Test+Gear (Autodesk Fusion 360 design; units mm, degrees)
Autodesk Fusion 360 part; units mm, degrees
sketch "Sketch1" plane through (0, 0, 0) normal (0, 0, 1) x (1, 0, 0) in component "Component"
  line L0 (0, 0) -> (2.9094, 11.25)
  line L1 (8.1773, 11.25) -> (11.0867, 0)
  line L2 (2.9094, 11.25) -> (8.1773, 11.25)
  line L3 (0, 0) -> (0, -10)
  line L4 (0, -10) -> (11.0867, -10)
  line L5 (11.0867, -10) -> (11.0867, 0)
  line L6 (6.3765, 0) -> (100, 0)
  line L7 (0, 0, 0) -> (0, 0, 10)
sketch "Sketch2" plane through (0, 0, 0) normal (0, 0, 1) x (1, 0, 0) in component "Component"
  line L0 (0, 0) -> (780.7769, 0)
  line L1 (0, 0) -> (0, -10)
  line L2 (0, -10) -> (780.7769, -10)
  line L3 (780.7769, -10) -> (780.7769, 0)
sweep "Sweep1" add kept parallel profiles "Sketch1" path "Sketch1" along L7 section 1 makes body 1 in component "Component"
pattern_path "PathPattern1" count 50 spacing 15.708 from (6.3765, 0, 0) path "Sketch1" along L6 of "Sweep1" makes body 2 makes body 3 makes body 4 makes body 5 makes body 6 makes body 7 makes body 8 makes body 9 makes body 10 makes body 11 makes body 12 makes body 13 makes body 14 makes body 15 makes body 16 makes body 17 makes body 18 makes body 19 makes body 20 makes body 21 makes body 22 makes body 23 makes body 24 makes body 25 makes body 26 makes body 27 makes body 28 makes body 29 makes body 30 makes body 31 makes body 32 makes body 33 makes body 34 makes body 35 makes body 36 makes body 37 makes body 38 makes body 39 makes body 40 makes body 41 makes body 42 makes body 43 makes body 44 makes body 45 makes body 46 makes body 47 makes body 48 makes body 49 makes body 50 in component "Component"
extrude "Extrude1" add sketch "Sketch2" along normal blind 10 bodies 1 2 3 4 5 6 7 8 9 10 11 12 13 14 15 16 17 18 19 20 21 22 23 24 25 26 27 28 29 30 31 32 33 34 35 36 37 38 39 40 41 42 43 44 45 46 47 48 49 50 in component "Component"
move_body "Move1" bodies 1 to x (1, 0, 0) y (0, 0, 1) z (0, -1, 0) at (0, -10, 10) in component "Component"
sketch "Sketch3" plane through (0, 0, 0) normal (0, 0, 1) x (1, 0, 0) in component "Component"
  line L0 (0, 0) -> (46.6318, 0) construction
  line L1 (46.6318, 0) -> (46.6318, 3) construction
  line L2 (46.6318, 3) -> (0, 3) construction
  line L3 (0, 3) -> (0, 0) construction
  constraint perpendicular L0 L1
  constraint parallel L0 L2
  constraint parallel L1 L3
sketch "Sketch1 (2)" plane through (0, 0, 0) normal (0, 0, 1) x (1, 0, 0) in component "Component'"
  spline S0 degree 5 poles (40.9519, -4.0239) (40.9523, -4.0239) (40.9533, -4.024) (40.9549, -4.0241) (40.9574, -4.0243) (40.9613, -4.0246) (40.9658, -4.0249) (40.9709, -4.0253) (40.9766, -4.0256) (40.9828, -4.026) (40.9896, -4.0264) (40.9968, -4.0268) (41.0046, -4.0271) (41.0128, -4.0275) (41.0215, -4.0279) (41.0307, -4.0282) (41.0402, -4.0285) (41.0502, -4.0288) (41.0606, -4.0291) (41.0714, -4.0293) (41.0825, -4.0295) (41.0941, -4.0297) (41.106, -4.0299) (41.1182, -4.03) (41.1308, -4.03) (41.1437, -4.0301) (41.157, -4.0301) (41.1705, -4.03) (41.1844, -4.0299) (41.1986, -4.0297) (41.2131, -4.0295) (41.2279, -4.0293) (41.243, -4.029) (41.2583, -4.0286) (41.274, -4.0282) (41.2899, -4.0278) (41.306, -4.0272) (41.3225, -4.0267) (41.3392, -4.026) (41.3561, -4.0253) (41.3733, -4.0246) (41.3908, -4.0237) (41.4084, -4.0228) (41.4264, -4.0219) (41.4445, -4.0209) (41.4629, -4.0198) (41.4815, -4.0187) (41.5003, -4.0174) (41.5194, -4.0162) (41.5386, -4.0148) (41.5581, -4.0134) (41.5778, -4.0119) (41.5977, -4.0103) (41.6178, -4.0087) (41.6381, -4.007) (41.6586, -4.0052) (41.6793, -4.0034) (41.7002, -4.0014) (41.7212, -3.9994) (41.7425, -3.9974) (41.764, -3.9952) (41.7856, -3.993) (41.8074, -3.9907) (41.8294, -3.9883) (41.8516, -3.9858) (41.8739, -3.9833) (41.8964, -3.9807) (41.9191, -3.978) (41.9419, -3.9752) (41.965, -3.9724) (41.9881, -3.9694) (42.0115, -3.9664) (42.035, -3.9633) (42.0586, -3.9602) (42.0825, -3.9569) (42.1064, -3.9536) (42.1305, -3.9501) (42.1548, -3.9466) (42.1792, -3.9431) (42.2038, -3.9394) (42.2285, -3.9356) (42.2534, -3.9318) (42.2784, -3.9279) (42.3036, -3.9239) (42.3289, -3.9198) (42.3543, -3.9156) (42.3799, -3.9113) (42.4056, -3.907) (42.4314, -3.9025) (42.4574, -3.898) (42.4835, -3.8934) (42.5097, -3.8887) (42.5361, -3.8839) (42.5626, -3.8791) (42.5892, -3.8741) (42.6159, -3.8691) (42.6428, -3.8639) (42.6698, -3.8587) (42.6969, -3.8534) (42.7241, -3.848) (42.7515, -3.8425) (42.779, -3.8369) (42.8066, -3.8313) (42.8343, -3.8255) (42.8621, -3.8197) (42.89, -3.8137) (42.9181, -3.8077) (42.9462, -3.8016) (42.9745, -3.7954) (43.0029, -3.7891) (43.0314, -3.7827) (43.06, -3.7762) (43.0887, -3.7696) (43.1175, -3.763) (43.1464, -3.7562) (43.1754, -3.7494) (43.2045, -3.7424) (43.2337, -3.7354) (43.2631, -3.7283) (43.2925, -3.7211) (43.322, -3.7138) (43.3516, -3.7064) (43.3814, -3.6989) (43.4112, -3.6913) (43.4411, -3.6836) (43.4711, -3.6759) (43.5012, -3.668) (43.5314, -3.66) (43.5617, -3.652) (43.592, -3.6438) (43.6225, -3.6356) (43.653, -3.6273) (43.6837, -3.6189) (43.7144, -3.6103) (43.7452, -3.6017) (43.7762, -3.593) (43.8071, -3.5842) (43.8382, -3.5753) (43.8694, -3.5663) (43.9006, -3.5573) (43.932, -3.5481) (43.9634, -3.5388) (43.9949, -3.5294) (44.0264, -3.52) (44.0581, -3.5104) (44.0898, -3.5008) (44.1216, -3.491) (44.1535, -3.4812) (44.1855, -3.4712) (44.2175, -3.4612) (44.2496, -3.4511) (44.2818, -3.4409) (44.3141, -3.4305) (44.3465, -3.4201) (44.3789, -3.4096) (44.4114, -3.399) (44.4439, -3.3883) (44.4765, -3.3775) (44.5093, -3.3666) (44.542, -3.3556) (44.5749, -3.3445) (44.6078, -3.3333) (44.6408, -3.3221) (44.6738, -3.3107) (44.7069, -3.2992) (44.7401, -3.2877) (44.7733, -3.276) (44.8067, -3.2642) (44.84, -3.2524) (44.8735, -3.2404) (44.907, -3.2284) (44.9405, -3.2162) (44.9742, -3.204) (45.0079, -3.1916) (45.0416, -3.1792) (45.0754, -3.1667) (45.1093, -3.154) (45.1432, -3.1413) (45.1772, -3.1285) (45.2113, -3.1156) (45.2454, -3.1025) (45.2795, -3.0894) (45.3138, -3.0762) (45.348, -3.0629) (45.3824, -3.0495) (45.4168, -3.036) (45.4512, -3.0224) (45.4857, -3.0087) (45.5203, -2.9949) (45.5549, -2.981) (45.5895, -2.967) (45.6242, -2.9529) (45.659, -2.9387) (45.6938, -2.9245) (45.7287, -2.9101) (45.7636, -2.8956) (45.7986, -2.881) (45.8336, -2.8664) (45.8687, -2.8516) (45.9038, -2.8367) (45.9389, -2.8218) (45.9741, -2.8067) (46.0094, -2.7915) (46.0447, -2.7763) (46.0801, -2.7609) (46.1154, -2.7455) (46.1509, -2.7299) (46.1864, -2.7143) (46.2219, -2.6985) (46.2575, -2.6827) (46.2931, -2.6668) (46.3288, -2.6507) (46.3645, -2.6346) (46.4002, -2.6184) (46.436, -2.602) (46.4718, -2.5856) (46.5077, -2.5691) (46.5436, -2.5525) (46.5796, -2.5357) (46.6155, -2.5189) (46.6516, -2.502) (46.6876, -2.485) (46.7237, -2.4679) (46.7599, -2.4507) (46.7961, -2.4334) (46.8323, -2.416) (46.8685, -2.3985) (46.9048, -2.3809) (46.9412, -2.3632) (46.9775, -2.3454) (47.0139, -2.3275) (47.0504, -2.3095) (47.0868, -2.2914) (47.1233, -2.2732) (47.1599, -2.255) (47.1964, -2.2366) (47.233, -2.2181) (47.2697, -2.1995) (47.3063, -2.1809) (47.343, -2.1621) (47.3798, -2.1432) (47.4092, -2.1281) (47.4312, -2.1166) (47.446, -2.109) (47.4533, -2.1052) knots 0 0 0 0 0 0 0.00416667 0.00833333 0.0125 0.01666667 0.02083333 0.025 0.02916667 0.03333333 0.0375 0.04166667 0.04583333 0.05 0.05416667 0.05833333 0.0625 0.06666667 0.07083333 0.075 0.07916667 0.08333333 0.0875 0.09166667 0.09583333 0.1 0.10416667 0.10833333 0.1125 0.11666667 0.12083333 0.125 0.12916667 0.13333333 0.1375 0.14166667 0.14583333 0.15 0.15416667 0.15833333 0.1625 0.16666667 0.17083333 0.175 0.17916667 0.18333333 0.1875 0.19166667 0.19583333 0.2 0.20416667 0.20833333 0.2125 0.21666667 0.22083333 0.225 0.22916667 0.23333333 0.2375 0.24166667 0.24583333 0.25 0.25416667 0.25833333 0.2625 0.26666667 0.27083333 0.275 0.27916667 0.28333333 0.2875 0.29166667 0.29583333 0.3 0.30416667 0.30833333 0.3125 0.31666667 0.32083333 0.325 0.32916667 0.33333333 0.3375 0.34166667 0.34583333 0.35 0.35416667 0.35833333 0.3625 0.36666667 0.37083333 0.375 0.37916667 0.38333333 0.3875 0.39166667 0.39583333 0.4 0.40416667 0.40833333 0.4125 0.41666667 0.42083333 0.425 0.42916667 0.43333333 0.4375 0.44166667 0.44583333 0.45 0.45416667 0.45833333 0.4625 0.46666667 0.47083333 0.475 0.47916667 0.48333333 0.4875 0.49166667 0.49583333 0.5 0.50416667 0.50833333 0.5125 0.51666667 0.52083333 0.525 0.52916667 0.53333333 0.5375 0.54166667 0.54583333 0.55 0.55416667 0.55833333 0.5625 0.56666667 0.57083333 0.575 0.57916667 0.58333333 0.5875 0.59166667 0.59583333 0.6 0.60416667 0.60833333 0.6125 0.61666667 0.62083333 0.625 0.62916667 0.63333333 0.6375 0.64166667 0.64583333 0.65 0.65416667 0.65833333 0.6625 0.66666667 0.67083333 0.675 0.67916667 0.68333333 0.6875 0.69166667 0.69583333 0.7 0.70416667 0.70833333 0.7125 0.71666667 0.72083333 0.725 0.72916667 0.73333333 0.7375 0.74166667 0.74583333 0.75 0.75416667 0.75833333 0.7625 0.76666667 0.77083333 0.775 0.77916667 0.78333333 0.7875 0.79166667 0.79583333 0.8 0.80416667 0.80833333 0.8125 0.81666667 0.82083333 0.825 0.82916667 0.83333333 0.8375 0.84166667 0.84583333 0.85 0.85416667 0.85833333 0.8625 0.86666667 0.87083333 0.875 0.87916667 0.88333333 0.8875 0.89166667 0.89583333 0.9 0.90416667 0.90833333 0.9125 0.91666667 0.92083333 0.925 0.92916667 0.93333333 0.9375 0.94166667 0.94583333 0.95 0.95416667 0.95833333 0.9625 0.96666667 0.97083333 0.975 0.97916667 0.98333333 0.9875 0.99166667 0.99583333 1 1 1 1 1 1
  spline S1 degree 5 poles (40.9519, 4.0239) (40.9523, 4.0239) (40.9533, 4.024) (40.9549, 4.0241) (40.9574, 4.0243) (40.9613, 4.0246) (40.9658, 4.0249) (40.9709, 4.0253) (40.9766, 4.0256) (40.9828, 4.026) (40.9896, 4.0264) (40.9968, 4.0268) (41.0046, 4.0271) (41.0128, 4.0275) (41.0215, 4.0279) (41.0307, 4.0282) (41.0402, 4.0285) (41.0502, 4.0288) (41.0606, 4.0291) (41.0714, 4.0293) (41.0825, 4.0295) (41.0941, 4.0297) (41.106, 4.0299) (41.1182, 4.03) (41.1308, 4.03) (41.1437, 4.0301) (41.157, 4.0301) (41.1705, 4.03) (41.1844, 4.0299) (41.1986, 4.0297) (41.2131, 4.0295) (41.2279, 4.0293) (41.243, 4.029) (41.2583, 4.0286) (41.274, 4.0282) (41.2899, 4.0278) (41.306, 4.0272) (41.3225, 4.0267) (41.3392, 4.026) (41.3561, 4.0253) (41.3733, 4.0246) (41.3908, 4.0237) (41.4084, 4.0228) (41.4264, 4.0219) (41.4445, 4.0209) (41.4629, 4.0198) (41.4815, 4.0187) (41.5003, 4.0174) (41.5194, 4.0162) (41.5386, 4.0148) (41.5581, 4.0134) (41.5778, 4.0119) (41.5977, 4.0103) (41.6178, 4.0087) (41.6381, 4.007) (41.6586, 4.0052) (41.6793, 4.0034) (41.7002, 4.0014) (41.7212, 3.9994) (41.7425, 3.9974) (41.764, 3.9952) (41.7856, 3.993) (41.8074, 3.9907) (41.8294, 3.9883) (41.8516, 3.9858) (41.8739, 3.9833) (41.8964, 3.9807) (41.9191, 3.978) (41.9419, 3.9752) (41.965, 3.9724) (41.9881, 3.9694) (42.0115, 3.9664) (42.035, 3.9633) (42.0586, 3.9602) (42.0825, 3.9569) (42.1064, 3.9536) (42.1305, 3.9501) (42.1548, 3.9466) (42.1792, 3.9431) (42.2038, 3.9394) (42.2285, 3.9356) (42.2534, 3.9318) (42.2784, 3.9279) (42.3036, 3.9239) (42.3289, 3.9198) (42.3543, 3.9156) (42.3799, 3.9113) (42.4056, 3.907) (42.4314, 3.9025) (42.4574, 3.898) (42.4835, 3.8934) (42.5097, 3.8887) (42.5361, 3.8839) (42.5626, 3.8791) (42.5892, 3.8741) (42.6159, 3.8691) (42.6428, 3.8639) (42.6698, 3.8587) (42.6969, 3.8534) (42.7241, 3.848) (42.7515, 3.8425) (42.779, 3.8369) (42.8066, 3.8313) (42.8343, 3.8255) (42.8621, 3.8197) (42.89, 3.8137) (42.9181, 3.8077) (42.9462, 3.8016) (42.9745, 3.7954) (43.0029, 3.7891) (43.0314, 3.7827) (43.06, 3.7762) (43.0887, 3.7696) (43.1175, 3.763) (43.1464, 3.7562) (43.1754, 3.7494) (43.2045, 3.7424) (43.2337, 3.7354) (43.2631, 3.7283) (43.2925, 3.7211) (43.322, 3.7138) (43.3516, 3.7064) (43.3814, 3.6989) (43.4112, 3.6913) (43.4411, 3.6836) (43.4711, 3.6759) (43.5012, 3.668) (43.5314, 3.66) (43.5617, 3.652) (43.592, 3.6438) (43.6225, 3.6356) (43.653, 3.6273) (43.6837, 3.6189) (43.7144, 3.6103) (43.7452, 3.6017) (43.7762, 3.593) (43.8071, 3.5842) (43.8382, 3.5753) (43.8694, 3.5663) (43.9006, 3.5573) (43.932, 3.5481) (43.9634, 3.5388) (43.9949, 3.5294) (44.0264, 3.52) (44.0581, 3.5104) (44.0898, 3.5008) (44.1216, 3.491) (44.1535, 3.4812) (44.1855, 3.4712) (44.2175, 3.4612) (44.2496, 3.4511) (44.2818, 3.4409) (44.3141, 3.4305) (44.3465, 3.4201) (44.3789, 3.4096) (44.4114, 3.399) (44.4439, 3.3883) (44.4765, 3.3775) (44.5093, 3.3666) (44.542, 3.3556) (44.5749, 3.3445) (44.6078, 3.3333) (44.6408, 3.3221) (44.6738, 3.3107) (44.7069, 3.2992) (44.7401, 3.2877) (44.7733, 3.276) (44.8067, 3.2642) (44.84, 3.2524) (44.8735, 3.2404) (44.907, 3.2284) (44.9405, 3.2162) (44.9742, 3.204) (45.0079, 3.1916) (45.0416, 3.1792) (45.0754, 3.1667) (45.1093, 3.154) (45.1432, 3.1413) (45.1772, 3.1285) (45.2113, 3.1156) (45.2454, 3.1025) (45.2795, 3.0894) (45.3138, 3.0762) (45.348, 3.0629) (45.3824, 3.0495) (45.4168, 3.036) (45.4512, 3.0224) (45.4857, 3.0087) (45.5203, 2.9949) (45.5549, 2.981) (45.5895, 2.967) (45.6242, 2.9529) (45.659, 2.9387) (45.6938, 2.9245) (45.7287, 2.9101) (45.7636, 2.8956) (45.7986, 2.881) (45.8336, 2.8664) (45.8687, 2.8516) (45.9038, 2.8367) (45.9389, 2.8218) (45.9741, 2.8067) (46.0094, 2.7915) (46.0447, 2.7763) (46.0801, 2.7609) (46.1154, 2.7455) (46.1509, 2.7299) (46.1864, 2.7143) (46.2219, 2.6985) (46.2575, 2.6827) (46.2931, 2.6668) (46.3288, 2.6507) (46.3645, 2.6346) (46.4002, 2.6184) (46.436, 2.602) (46.4718, 2.5856) (46.5077, 2.5691) (46.5436, 2.5525) (46.5796, 2.5357) (46.6155, 2.5189) (46.6516, 2.502) (46.6876, 2.485) (46.7237, 2.4679) (46.7599, 2.4507) (46.7961, 2.4334) (46.8323, 2.416) (46.8685, 2.3985) (46.9048, 2.3809) (46.9412, 2.3632) (46.9775, 2.3454) (47.0139, 2.3275) (47.0504, 2.3095) (47.0868, 2.2914) (47.1233, 2.2732) (47.1599, 2.255) (47.1964, 2.2366) (47.233, 2.2181) (47.2697, 2.1995) (47.3063, 2.1809) (47.343, 2.1621) (47.3798, 2.1432) (47.4092, 2.1281) (47.4312, 2.1166) (47.446, 2.109) (47.4533, 2.1052) knots 0 0 0 0 0 0 0.00416667 0.00833333 0.0125 0.01666667 0.02083333 0.025 0.02916667 0.03333333 0.0375 0.04166667 0.04583333 0.05 0.05416667 0.05833333 0.0625 0.06666667 0.07083333 0.075 0.07916667 0.08333333 0.0875 0.09166667 0.09583333 0.1 0.10416667 0.10833333 0.1125 0.11666667 0.12083333 0.125 0.12916667 0.13333333 0.1375 0.14166667 0.14583333 0.15 0.15416667 0.15833333 0.1625 0.16666667 0.17083333 0.175 0.17916667 0.18333333 0.1875 0.19166667 0.19583333 0.2 0.20416667 0.20833333 0.2125 0.21666667 0.22083333 0.225 0.22916667 0.23333333 0.2375 0.24166667 0.24583333 0.25 0.25416667 0.25833333 0.2625 0.26666667 0.27083333 0.275 0.27916667 0.28333333 0.2875 0.29166667 0.29583333 0.3 0.30416667 0.30833333 0.3125 0.31666667 0.32083333 0.325 0.32916667 0.33333333 0.3375 0.34166667 0.34583333 0.35 0.35416667 0.35833333 0.3625 0.36666667 0.37083333 0.375 0.37916667 0.38333333 0.3875 0.39166667 0.39583333 0.4 0.40416667 0.40833333 0.4125 0.41666667 0.42083333 0.425 0.42916667 0.43333333 0.4375 0.44166667 0.44583333 0.45 0.45416667 0.45833333 0.4625 0.46666667 0.47083333 0.475 0.47916667 0.48333333 0.4875 0.49166667 0.49583333 0.5 0.50416667 0.50833333 0.5125 0.51666667 0.52083333 0.525 0.52916667 0.53333333 0.5375 0.54166667 0.54583333 0.55 0.55416667 0.55833333 0.5625 0.56666667 0.57083333 0.575 0.57916667 0.58333333 0.5875 0.59166667 0.59583333 0.6 0.60416667 0.60833333 0.6125 0.61666667 0.62083333 0.625 0.62916667 0.63333333 0.6375 0.64166667 0.64583333 0.65 0.65416667 0.65833333 0.6625 0.66666667 0.67083333 0.675 0.67916667 0.68333333 0.6875 0.69166667 0.69583333 0.7 0.70416667 0.70833333 0.7125 0.71666667 0.72083333 0.725 0.72916667 0.73333333 0.7375 0.74166667 0.74583333 0.75 0.75416667 0.75833333 0.7625 0.76666667 0.77083333 0.775 0.77916667 0.78333333 0.7875 0.79166667 0.79583333 0.8 0.80416667 0.80833333 0.8125 0.81666667 0.82083333 0.825 0.82916667 0.83333333 0.8375 0.84166667 0.84583333 0.85 0.85416667 0.85833333 0.8625 0.86666667 0.87083333 0.875 0.87916667 0.88333333 0.8875 0.89166667 0.89583333 0.9 0.90416667 0.90833333 0.9125 0.91666667 0.92083333 0.925 0.92916667 0.93333333 0.9375 0.94166667 0.94583333 0.95 0.95416667 0.95833333 0.9625 0.96666667 0.97083333 0.975 0.97916667 0.98333333 0.9875 0.99166667 0.99583333 1 1 1 1 1 1
  spline S2 degree 5 poles (40.9491, -4.0236) (40.9492, -4.0236) (40.9494, -4.0236) (40.9498, -4.0237) (40.9502, -4.0237) (40.9508, -4.0238) (40.9512, -4.0238) (40.9516, -4.0238) (40.9518, -4.0239) (40.9519, -4.0239) knots 0 0 0 0 0 0 0.2 0.4 0.6 0.8 1 1 1 1 1 1
  spline S3 degree 5 poles (40.9491, 4.0236) (40.9492, 4.0236) (40.9494, 4.0236) (40.9498, 4.0237) (40.9502, 4.0237) (40.9508, 4.0238) (40.9512, 4.0238) (40.9516, 4.0238) (40.9518, 4.0239) (40.9519, 4.0239) knots 0 0 0 0 0 0 0.2 0.4 0.6 0.8 1 1 1 1 1 1
  line L0 (0, 0) -> (40.9491, -4.0236)
  line L1 (0, 0) -> (40.9491, 4.0236)
  arc A0 (47.4533, -2.1052) -> (47.4533, 2.1052) centre (0, 0) ccw
  point P0 (40.9604, -4.0246)
  point P1 (40.9747, -4.0255)
  point P2 (40.9946, -4.0266)
  point P3 (41.0202, -4.0278)
  point P4 (41.0515, -4.0288)
  point P5 (41.0886, -4.0296)
  point P6 (41.1314, -4.03)
  point P7 (41.1798, -4.0299)
  point P8 (41.234, -4.0292)
  point P9 (41.2938, -4.0276)
  point P10 (41.3593, -4.0252)
  point P11 (41.4305, -4.0217)
  point P12 (41.5073, -4.017)
  point P13 (41.5898, -4.0109)
  point P14 (41.6778, -4.0035)
  point P15 (41.7715, -3.9944)
  point P16 (41.8706, -3.9837)
  point P17 (41.9754, -3.9711)
  point P18 (42.0856, -3.9565)
  point P19 (42.2012, -3.9398)
  point P20 (42.3224, -3.9208)
  point P21 (42.4488, -3.8995)
  point P22 (42.5807, -3.8757)
  point P23 (42.7178, -3.8492)
  point P24 (42.8603, -3.82)
  point P25 (43.0079, -3.7879)
  point P26 (43.1607, -3.7528)
  point P27 (43.3186, -3.7146)
  point P28 (43.4816, -3.6731)
  point P29 (43.6496, -3.6282)
  point P30 (43.8225, -3.5798)
  point P31 (44.0004, -3.5278)
  point P32 (44.183, -3.472)
  point P33 (44.3704, -3.4123)
  point P34 (44.5626, -3.3487)
  point P35 (44.7593, -3.2809)
  point P36 (44.9606, -3.2089)
  point P37 (45.1664, -3.1325)
  point P38 (45.3766, -3.0517)
  point P39 (45.5911, -2.9663)
  point P40 (45.8099, -2.8763)
  point P41 (46.0329, -2.7814)
  point P42 (46.2599, -2.6816)
  point P43 (46.4909, -2.5768)
  point P44 (46.7259, -2.4668)
  point P45 (46.9647, -2.3517)
  point P46 (47.2072, -2.2312)
  point P47 (40.9604, 4.0246)
  point P48 (40.9747, 4.0255)
  point P49 (40.9946, 4.0266)
  point P50 (41.0202, 4.0278)
  point P51 (41.0515, 4.0288)
  point P52 (41.0886, 4.0296)
  point P53 (41.1314, 4.03)
  point P54 (41.1798, 4.0299)
  point P55 (41.234, 4.0292)
  point P56 (41.2938, 4.0276)
  point P57 (41.3593, 4.0252)
  point P58 (41.4305, 4.0217)
  point P59 (41.5073, 4.017)
  point P60 (41.5898, 4.0109)
  point P61 (41.6778, 4.0035)
  point P62 (41.7715, 3.9944)
  point P63 (41.8706, 3.9837)
  point P64 (41.9754, 3.9711)
  point P65 (42.0856, 3.9565)
  point P66 (42.2012, 3.9398)
  point P67 (42.3224, 3.9208)
  point P68 (42.4488, 3.8995)
  point P69 (42.5807, 3.8757)
  point P70 (42.7178, 3.8492)
  point P71 (42.8603, 3.82)
  point P72 (43.0079, 3.7879)
  point P73 (43.1607, 3.7528)
  point P74 (43.3186, 3.7146)
  point P75 (43.4816, 3.6731)
  point P76 (43.6496, 3.6282)
  point P77 (43.8225, 3.5798)
  point P78 (44.0004, 3.5278)
  point P79 (44.183, 3.472)
  point P80 (44.3704, 3.4123)
  point P81 (44.5626, 3.3487)
  point P82 (44.7593, 3.2809)
  point P83 (44.9606, 3.2089)
  point P84 (45.1664, 3.1325)
  point P85 (45.3766, 3.0517)
  point P86 (45.5911, 2.9663)
  point P87 (45.8099, 2.8763)
  point P88 (46.0329, 2.7814)
  point P89 (46.2599, 2.6816)
  point P90 (46.4909, 2.5768)
  point P91 (46.7259, 2.4668)
  point P92 (46.9647, 2.3517)
  point P93 (47.2072, 2.2312)
sketch "Sketch2 (2)" plane through (0, 0, 0) normal (0, 0, 1) x (1, 0, 0) in component "Component'"
  circle A0 centre (0, 0) radius 36.25
extrude "Extrude1'" add sketch "Sketch2 (2)" along normal blind 10 separate body makes body 51 in component "Component'"
extrude "Extrude2" add sketch "Sketch1 (2)" along normal blind 10 separate body makes body 52 in component "Component'"
pattern_circular "C-Pattern1" count 17 over 360 about axis through (0, 0, 1.75) along (0, 0, 1) of "Extrude2" makes body 53 makes body 54 makes body 55 makes body 56 makes body 57 makes body 58 makes body 59 makes body 60 makes body 61 makes body 62 makes body 63 makes body 64 makes body 65 makes body 66 makes body 67 makes body 68 in component "Component'"
combine "Combine1" operation add target body 51 tool bodies 52 53 54 55 56 57 58 59 60 61 62 63 64 65 66 67 68 in component "Component'"
sketch "Sketch3 (2)" plane through (0, 0, 0) normal (0, 0, 1) x (1, 0, 0) in component "Component'"
  line L0 (0, 0) -> (46.6465, 0) construction
  line L1 (46.6465, 0) -> (46.6465, 3) construction
  line L2 (46.6465, 3) -> (0, 3) construction
  line L3 (0, 3) -> (0, 0) construction
  constraint perpendicular L0 L1
  constraint parallel L0 L2
  constraint parallel L1 L3
component "Component" placed x (1, 0, 0) y (0, 1, 0) z (0, 0, 1) at (0, 0, 0)
component "Component'" placed x (1, 0, 0) y (0, 1, 0) z (0, 0, 1) at (0, 0, 0)
